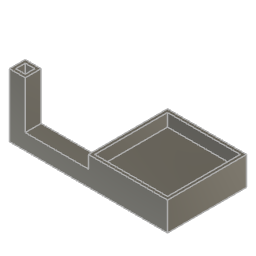
metunus_корпус (Autodesk Fusion 360 design; units mm, degrees)
Autodesk Fusion 360 part; units mm, degrees
sketch "Sketch1" plane through (0, 0, 0) normal (0, 0, 1) x (1, 0, 0)
  line L0 (0, 0) -> (25, 0)
  line L1 (25, 0) -> (25, 25)
  line L2 (25, 25) -> (0, 25)
  line L3 (0, 25) -> (0, 5)
  line L4 (0, 0) -> (-20, 0)
  line L5 (-20, 0) -> (-20, 5)
  line L6 (-20, 5) -> (0, 5)
  constraint coincident L0.start L4.start
  constraint horizontal L0
  constraint perpendicular L0 L1
  constraint perpendicular L1 L2
  constraint perpendicular L0 L3
  constraint perpendicular L3 L4
  constraint perpendicular L4 L5
  constraint perpendicular L3 L6
extrude "Extrude1" add sketch "Sketch1" along normal blind 1
sketch "Sketch2" plane through (0, 0, 1) normal (0, 0, 1) x (-1, 0, 0)
  line L0 (20, 0) -> (-25, 0)
  line L1 (-25, 0) -> (-25, -25)
  line L2 (-25, -25) -> (0, -25)
  line L3 (0, -25) -> (0, -5)
  line L4 (0, -5) -> (20, -5)
  line L5 (20, -5) -> (20, 0)
  line L6 (-1, -1) -> (-24, -1)
  line L7 (-24, -1) -> (-24, -24)
  line L8 (-24, -24) -> (-1, -24)
  line L9 (-1, -24) -> (-1, -1)
  line L10 (0, -5) -> (0, 0)
  constraint perpendicular L1 L6
  constraint perpendicular L6 L7
  constraint perpendicular L7 L8
  constraint perpendicular L8 L9
  constraint coincident L3.end L4.start
  constraint coincident L10.end origin
extrude "Extrude2" add sketch "Sketch2" along normal blind 4
sketch "Sketch3" plane through (0, 0, 5) normal (0, 0, 1) x (-1, 0, 0)
  line L0 (-1, -1) -> (-1, -24)
  line L1 (-1, -24) -> (-24, -24)
  line L2 (-24, -24) -> (-24, -1)
  line L3 (-24, -1) -> (-1, -1)
  line L4 (20, -5) -> (20, 0)
  line L5 (20, 0) -> (-25, 0)
  line L6 (-25, 0) -> (-25, -25)
  line L7 (-25, -25) -> (0, -25)
  line L8 (0, -25) -> (0, -5)
  line L9 (0, -5) -> (20, -5)
  line L10 (0, -5) -> (0, 0)
  constraint coincident L8.end L9.start
  constraint coincident L10.end origin
extrude "Extrude3" add sketch "Sketch3" along normal blind 10 contours L5 L6 L7 L8 L10
sketch "Sketch4" plane through (-20, 0, 0) normal (-1, 0, 0) x (0, -1, 0)
  line L0 (-5, 0) -> (0, 0)
  line L1 (0, 0) -> (0, 5)
  line L2 (0, 5) -> (-5, 5)
  line L3 (-5, 5) -> (-5, 0)
  line L4 (-4, 4) -> (-1, 4)
  line L5 (-1, 4) -> (-1, 1)
  line L6 (-1, 1) -> (-4, 1)
  line L7 (-4, 1) -> (-4, 4)
  constraint perpendicular L1 L4
  constraint perpendicular L4 L5
  constraint perpendicular L1 L6
  constraint perpendicular L4 L7
extrude "Extrude4" cut sketch "Sketch4" against normal blind 23 contours L4 L5 L6 L7
sketch "Sketch5" plane through (0, 1, 0) normal (0, 1, 0) x (-1, 0, 0)
  line L0 (-24, 1) -> (20, 1)
  line L1 (20, 1) -> (20, 4)
  line L2 (20, 4) -> (-1, 4)
  line L3 (-1, 4) -> (-1, 15)
  line L4 (-1, 15) -> (-24, 15)
  line L5 (-24, 15) -> (-24, 1)
  line L6 (-1, 4) -> (-24, 4)
  line L7 (-24, 4) -> (-24, 5)
  line L8 (-24, 5) -> (-1, 5)
  line L9 (-1, 4) -> (-1, 5)
  constraint coincident L2.end L3.start
  constraint coincident L5 L6.end
  constraint perpendicular L5 L6
  constraint coincident L5 L7.end
  constraint coincident L3 L8.end
  constraint perpendicular L3 L8
extrude "Extrude5" add sketch "Sketch5" along normal blind 23 contours L3 L5 L6 L7 L8 L9
sketch "Sketch6" plane through (0, 5, 0) normal (0, 1, 0) x (-1, 0, 0)
  line L0 (0, 0) -> (20, 0)
  line L1 (20, 0) -> (20, 5)
  line L2 (20, 5) -> (0, 5)
  line L3 (0, 5) -> (0, 0)
  line L4 (0, 4) -> (1.5, 4)
  line L5 (1.5, 4) -> (1.5, 2.5)
  line L6 (1.5, 2.5) -> (0, 2.5)
  line L7 (0, 4) -> (0, 2.5)
  constraint coincident L3 L4.start
  constraint perpendicular L3 L4
  constraint perpendicular L0 L5
  constraint midpoint L3 L6.end
  constraint perpendicular L3 L6
extrude "Extrude6" cut sketch "Sketch6" against normal blind 2 contours L3 L4 L5 L6 L7
sketch "Sketch7" plane through (-20, 0, 0) normal (-1, 0, 0) x (0, -1, 0)
  line L0 (-1, 4) -> (-1, 1)
  line L1 (-1, 1) -> (-4, 1)
  line L2 (-4, 1) -> (-4, 4)
  line L3 (-4, 4) -> (-1, 4)
  line L4 (-5, 0) -> (0, 0)
  line L5 (0, 0) -> (0, 5)
  line L6 (0, 5) -> (-5, 5)
  line L7 (-5, 5) -> (-5, 0)
  line L8 (-5, 1) -> (0, 1)
  constraint coincident L7 L8.start
  constraint coincident L5 L8.end
  constraint perpendicular L5 L8
extrude "Extrude7" add sketch "Sketch7" along normal blind 6 contours L1 L4 L5 L7 L8
sketch "Sketch8" plane through (0, 0, 1) normal (0, 0, 1) x (-1, 0, 0)
  line L0 (20, -1) -> (-24, -1)
  line L1 (-24, -1) -> (-24, -24)
  line L2 (-24, -24) -> (-1, -24)
  line L3 (-1, -24) -> (-1, -4)
  line L4 (-1, -4) -> (20, -4)
  line L5 (20, -4) -> (20, -5)
  line L6 (20, -5) -> (26, -5)
  line L7 (26, -5) -> (26, 0)
  line L8 (26, 0) -> (20, 0)
  line L9 (20, 0) -> (20, -1)
  line L10 (20, -1) -> (24, -1)
  line L11 (24, -1) -> (24, -4)
  line L12 (24, -4) -> (20, -4)
  constraint coincident L0.start L9.end
  constraint perpendicular L9 L10
  constraint perpendicular L10 L11
  constraint coincident L4.end L5.start
  constraint perpendicular L5 L12
extrude "Extrude8" add sketch "Sketch8" along normal blind 4 contours L5 L6 L7 L8 L9 L10 L11 L12
extrude "Extrude9" cut 1 faces at (-26, 3.3333, 1.6667) along direction (1, 0, 0) blind 1
extrude "Extrude10" add 1 faces at (-20, 2, 4.3333) along direction (-1, 0, 0) blind 1
sketch "Sketch9" plane through (0, 0, 5) normal (0, 0, 1) x (-1, 0, 0)
  line L0 (21, -1) -> (24, -1)
  line L1 (24, -1) -> (24, -4)
  line L2 (24, -4) -> (21, -4)
  line L3 (21, -4) -> (21, -1)
  line L4 (25, -5) -> (25, 0)
  line L5 (25, 0) -> (0, 0)
  line L6 (0, 0) -> (0, -5)
  line L7 (0, -5) -> (25, -5)
  line L8 (20, 0) -> (20, -5)
  constraint coincident L5 L8.start
  constraint coincident L7 L8.end
  constraint perpendicular L7 L8
extrude "Extrude11" add sketch "Sketch9" along normal blind 15 contours L4 L5 L7 L8
extrude "Extrude12" cut 1 faces at (16.3333, 0.3333, 15) along direction (0, 0, -1) blind 6
